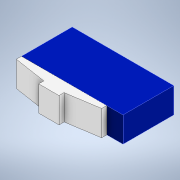
# Autodesk Inventor part: Switch_ESP2010_90
Saved by Autodesk Inventor 2021 (Build 250183000, 183)
## iProperties
Created: 2021-07-22
Part Number: Switch_ESP2010_90
Material: Generic
Document SubType Name: Modeling
Designer: ermoz
Density: 1 g/cm^3
Appearance: Default
Author: ermoz
Autodesk Inventor part; units mm, degrees
ref_plane "YZ Plane" through (0, 0, 0) normal (1, 0, 0) x (0, 1, 0)
ref_plane "XZ Plane" through (0, 0, 0) normal (0, 1, 0) x (-1, 0, 0)
ref_plane "XY Plane" through (0, 0, 0) normal (0, 0, 1) x (1, 0, 0)
sketch "Sketch1" plane through (0, 0, 0) normal (0, 1, 0) x (-1, 0, 0)
  line L0 (5, -2.5) -> (-5, -2.5)
  line L1 (-5, -2.5) -> (-5, 2.5)
  line L2 (-5, 2.5) -> (5, 2.5)
  line L3 (5, 2.5) -> (5, -2.5)
  line L4 (5, -2.5) -> (-5, 2.5) construction
  line L5 (-5, -2.5) -> (5, 2.5) construction
  point P0 (0, 0)
  dimension "d0" = 10
  dimension "d1" = 5
  constraints: 12 end point, 2 midpoint, 2 parallel, 1 horizontal, 1 perpendicular
  measures "d0" distance of L1.end L2.end
  measures "d1" distance of L0.end L1.end
extrude "Extrusion1" add sketch "Sketch1" along normal blind 2.5
sketch "Sketch2" plane through (-5, 0, 2.5) normal (0, 0, 1) x (1, 0, 0)
  line L0 (0, 2.5) -> (10, 2.5) projected
  line L1 (0, 0) -> (10, 0) projected
  line L2 (0, 2.5) -> (8.4, 2.5)
  line L3 (8.4, 2.5) -> (8.4, 0)
  line L4 (8.4, 0) -> (0, 0)
  line L5 (0, 0) -> (0, 2.5)
  point P0 (5, 0)
  dimension "d4" = 8.4
  constraints: 8 end point, 2 parallel, 1 horizontal, 1 perpendicular, 1 point on line
  measures "d4" distance of L3.end L4.end
extrude "Extrusion2" add sketch "Sketch2" along normal blind 1.5 separate body
sketch "Sketch3" plane through (-5, 0, 2.5) normal (0, -1, 0) x (1, 0, 0)
  line L0 (0, 1.5) -> (8.4, 1.5) projected
  line L1 (3.2, 1.5) -> (5.2, 1.5)
  line L2 (5.2, 1.5) -> (5.2, 1)
  line L3 (5.2, 1) -> (3.2, 1)
  line L4 (3.2, 1) -> (3.2, 1.5)
  line L5 (0, 0) -> (10, 0) projected
  line L6 (8.4, 0) -> (8.4, 1.5) projected
  line L7 (0, 0) -> (8.4, 0)
  line L8 (8.4, 0) -> (8.4, 0.5)
  line L9 (8.4, 0.5) -> (0, 0.5)
  line L10 (0, 0.5) -> (0, 0)
  line L11 (3.2, 1) -> (0, 0.5)
  line L12 (5.2, 1) -> (8.4, 0.5)
  line L13 (0, 1.5) -> (8.4, 1.5)
  line L14 (8.4, 1.5) -> (8.4, 0)
  line L15 (8.4, 0) -> (0, 0)
  line L16 (0, 0) -> (0, 1.5)
  point P0 (5, -2.5)
  point P1 (0, 0.5)
  dimension "d7" = 2
  dimension "d8" = 0.5
  dimension "d9" = 0.5
  constraints: 28 end point, 6 parallel, 3 horizontal, 3 perpendicular, 2 point on line, 1 equal length
  measures "d7" distance between parallel lines of L4 L2
  measures "d8" distance of L9.end L5.start
  measures "d9" distance of L3.end L1.start
extrude "Extrusion3" cut sketch "Sketch3" against normal through all contours L0 L4 L11 L16 | L0 L6 L12 L2 bodies 2
body "Solid1"
body "Solid2"
